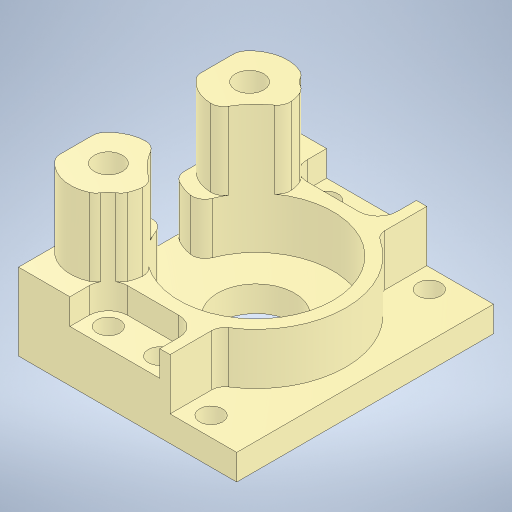
# Autodesk Inventor part: Spring Mount
Saved by Autodesk Inventor 2023.2 (Build 272271000, 271)
## iProperties
Created: 2024-03-24
Part Number: Spring Mount
Material: Nylon 6/6
Document SubType Name: Modeling
Designer: Nathan Cai
Density: 1.13 g/cm^3
Appearance: Nylon 6
Author: Nathan Cai
Autodesk Inventor part; units mm, degrees
ref_plane "YZ Plane" through (0, 0, 0) normal (1, 0, 0) x (0, 1, 0)
ref_plane "XZ Plane" through (0, 0, 0) normal (0, 1, 0) x (-1, 0, 0)
ref_plane "XY Plane" through (0, 0, 0) normal (0, 0, 1) x (1, 0, 0)
sketch "Sketch1" plane through (0, 0, 0) normal (0, 1, 0) x (-1, 0, 0)
  line L0 (-13.4938, 15.875) -> (13.4937, 15.875)
  line L1 (13.4937, 15.875) -> (13.4937, -15.875)
  line L2 (13.4937, -15.875) -> (-13.4938, -15.875)
  line L3 (-13.4938, -15.875) -> (-13.4938, 15.875)
  line L4 (-13.4938, 15.875) -> (13.4937, -15.875) construction
  line L5 (13.4937, 15.875) -> (-13.4938, -15.875) construction
  circle A0 centre (0, 0) radius 4.7625
  circle A1 centre (9.525, 8.7313) radius 6.35 construction
  line L6 (13.4937, 0) -> (-13.4938, 0) construction
  circle A2 centre (9.525, 8.7313) radius 1.7526
  circle A3 centre (9.525, -8.7312) radius 6.35 construction
  circle A4 centre (9.525, -8.7312) radius 1.7526
  dimension "d0" = 26.9875
  dimension "d1" = 31.75
  dimension "d2" = 9.525
  dimension "d3" = 12.7
  dimension "d4" = 3.5052
  dimension "d7" = 8.7312
  dimension "d8" = 3.9688
  constraints: 14 end point, 5 centre point, 4 midpoint, 2 coincident, 2 parallel, 2 symmetric about line, 1 horizontal, 1 perpendicular, 2 other
  measures "d0" distance of L1.end L2.end
  measures "d1" distance of L0.end L1.end
  measures "d2" diameter of A0
  measures "d3" diameter of A1
  measures "d4" diameter of A2
  measures "d7" distance from line of L6 A2.centre
  measures "d8" distance from line of L1 A2.centre
extrude "Extrusion1" add sketch "Sketch1" along normal blind 3.175
sketch "Sketch2" plane through (0, 3.175, 0) normal (0, 1, 0) x (1, 0, 0)
  circle A0 centre (0, 0) radius 9.525
  circle A1 centre (-9.525, 8.7312) radius 1.7526 projected
  circle A2 centre (-9.525, 8.7312) radius 6.35
  line L0 (13.4938, 15.875) -> (-13.4937, 15.875) projected
  line L1 (-13.4937, 15.875) -> (-13.4937, -15.875) projected
  line L2 (-13.4937, -15.875) -> (13.4938, -15.875) projected
  line L3 (13.4938, -15.875) -> (13.4938, 15.875) projected
  circle A3 centre (-9.525, 8.7312) radius 1.7526 projected
  circle A4 centre (-9.525, -8.7313) radius 1.7526 projected
  circle A5 centre (0, 0) radius 4.7625 projected
  circle A6 centre (-9.525, -8.7313) radius 6.35
  point P0 (-13.4937, 13.6882)
  point P1 (-13.4937, 3.7743)
  point P2 (-9.2207, 2.3885)
  point P3 (-3.1798, 8.9786)
  point P4 (-9.2207, -2.3885)
  point P5 (-13.4937, -3.7743)
  point P6 (-13.4937, -13.6882)
  point P7 (-3.1798, -8.9786)
  dimension "d9" = 19.05
  dimension "d10" = 12.7
  dimension "d11" = 12.7
  constraints: 3 centre point, 3 coincident
  measures "d9" diameter of A0
  measures "d10" diameter of A2
  measures "d11" diameter of A6
extrude "Extrusion2" add sketch "Sketch2" along normal blind 6.35 contours A0 A2 L1 L0 L3 L2 A6 | A0 A2 L1 | A6 L1 A0
sketch "Sketch3" plane through (0, 9.525, 0) normal (0, 1, 0) x (1, 0, 0)
  circle A0 centre (-9.525, -8.7313) radius 1.7526 projected
  circle A1 centre (-9.525, -8.7313) radius 4.699
  circle A2 centre (-9.525, 8.7312) radius 1.7526 projected
  circle A3 centre (-9.525, 8.7312) radius 4.699
  arc A4 (-13.4937, 3.7743) -> (-9.2207, 2.3885) centre (-9.525, 8.7312) ccw projected
  arc A5 (-9.2207, -2.3885) -> (-9.2207, 2.3885) centre (0, 0) ccw projected
  line L0 (-13.4937, 15.875) -> (-13.4937, 3.7743) projected
  circle A6 centre (-9.525, 8.7312) radius 1.7526 projected
  line L1 (-13.4937, -3.7743) -> (-13.4937, -15.875) projected
  arc A7 (-9.2207, -2.3885) -> (-13.4937, -3.7743) centre (-9.525, -8.7313) ccw projected
  arc A8 (-9.2207, -2.3885) -> (-9.2207, 2.3885) centre (0, 0) ccw projected
  circle A9 centre (-9.525, -8.7313) radius 1.7526 projected
  arc A10 (-13.4937, 3.7743) -> (-9.2207, 2.3885) centre (-9.525, 8.7312) ccw projected
  line L2 (-13.4937, -15.875) -> (13.4938, -15.875) projected
  line L3 (13.4938, -15.875) -> (13.4938, 15.875) projected
  line L4 (13.4938, 15.875) -> (-13.4937, 15.875) projected
  line L5 (-13.4937, 15.875) -> (-13.4937, 3.7743) projected
  arc A11 (-9.2207, -2.3885) -> (-13.4937, -3.7743) centre (-9.525, -8.7313) ccw projected
  line L6 (-13.4937, -3.7743) -> (-13.4937, -15.875) projected
  line L7 (-13.4937, -15.875) -> (13.4938, -15.875) projected
  line L8 (13.4938, -15.875) -> (13.4938, 15.875) projected
  line L9 (13.4938, 15.875) -> (-13.4937, 15.875) projected
  point P0 (-4.8568, -8.1937)
  point P1 (-8.5843, -4.1274)
  point P2 (-13.4937, -6.2154)
  point P3 (-13.4937, -11.2471)
  point P4 (-13.4937, 11.2471)
  point P5 (-13.4937, 6.2154)
  point P6 (-8.5843, 4.1274)
  point P7 (-4.8568, 8.1937)
  dimension "d14" = 9.398
  dimension "d15" = 9.398
  constraints: 2 centre point, 2 coincident
  measures "d14" diameter of A1
  measures "d15" diameter of A3
extrude "Extrusion3" add sketch "Sketch3" along normal blind 9.525 contours A1 L1 A5 | A5 A3 L0
sketch "Sketch4" plane through (0, 0, 0) normal (0, -1, 0) x (1, 0, 0)
  line L0 (-13.4937, -3.7743) -> (-13.4937, 3.7743) projected
  line L1 (-13.4937, 13.4938) -> (13.4938, 13.4937) construction
  line L2 (13.4938, 15.875) -> (13.4938, -15.875) projected
  line L3 (-13.4937, 15.875) -> (13.4938, 15.875) projected
  circle A0 centre (-11.1125, 13.4938) radius 1.4224
  circle A1 centre (-4.7625, 13.4937) radius 1.4224
  circle A2 centre (1.5875, 13.4937) radius 1.4224
  circle A3 centre (7.9375, 13.4937) radius 1.4224
  line L4 (-13.4937, -3.7743) -> (-13.4937, 3.7743) projected
  line L5 (-13.4937, 0) -> (13.4938, 0) construction
  line L6 (-13.4938, -13.4937) -> (13.4938, -13.4937) construction
  circle A4 centre (-11.1125, -13.4937) radius 1.4224
  circle A5 centre (-4.7625, -13.4937) radius 1.4224
  circle A6 centre (1.5875, -13.4937) radius 1.4224
  circle A7 centre (7.9375, -13.4937) radius 1.4224
  point P0 (0, 0)
  point P1 (-13.4937, 12.8557)
  point P2 (-13.4937, -4.6068)
  point P3 (-13.4937, 4.6068)
  dimension "d19" = 2.3813
  dimension "d20" = 2.8448
  dimension "d21" = 2.3813
  dimension "d24" = 6.35
  constraints: 8 centre point, 6 end point, 6 symmetric about line, 4 point on line, 2 midpoint, 1 horizontal, 1 parallel, 10 other
  measures "d19" distance between parallel lines of L3 L1
  measures "d20" diameter of A0
  measures "d21" distance from line of L0 A0.centre
  measures "d24" distance of A0.centre A1.centre
extrude "Extrusion4" cut sketch "Sketch4" against normal blind 6.35
sketch "Sketch5" plane through (0, 9.525, 0) normal (0, 1, 0) x (1, 0, 0)
  circle A0 centre (7.9375, -13.4937) radius 1.4224 projected
  line L0 (13.4938, -15.875) -> (13.4938, 15.875) projected
  line L1 (13.4938, 0) -> (-13.4937, 0) construction
  line L2 (-13.4937, 15.875) -> (-13.4937, -15.875) projected
  circle A1 centre (1.5875, -13.4937) radius 1.4224 projected
  circle A2 centre (-4.7625, -13.4937) radius 1.4224 projected
  line L3 (1.5875, -13.4937) -> (-4.7625, -13.4937) construction
  line L4 (1.5875, -11.1125) -> (-4.7625, -11.1125)
  line L5 (-4.7625, -15.875) -> (1.5875, -15.875)
  arc A3 (1.5875, -15.875) -> (1.5875, -11.1125) centre (1.5875, -13.4937) ccw
  arc A4 (-4.7625, -11.1125) -> (-4.7625, -15.875) centre (-4.7625, -13.4937) ccw
  line L6 (-13.4937, -15.875) -> (13.4938, -15.875) projected
  line L7 (3.9688, -13.4937) -> (-7.1437, -13.4937) construction
  line L8 (-7.1437, -13.4937) -> (-7.1437, -15.875)
  line L9 (-7.1437, -15.875) -> (3.9688, -15.875)
  line L10 (3.9688, -15.875) -> (3.9688, -13.4937)
  circle A5 centre (1.5875, 13.4937) radius 1.4224
  circle A6 centre (-4.7625, 13.4937) radius 1.4224
  line L11 (1.5875, 13.4937) -> (-4.7625, 13.4937) construction
  line L12 (1.5875, 11.1125) -> (-4.7625, 11.1125)
  line L13 (-4.7625, 15.875) -> (1.5875, 15.875)
  arc A7 (1.5875, 11.1125) -> (1.5875, 15.875) centre (1.5875, 13.4937) ccw
  arc A8 (-4.7625, 15.875) -> (-4.7625, 11.1125) centre (-4.7625, 13.4937) ccw
  line L14 (3.9688, 13.4937) -> (-7.1437, 13.4937) construction
  line L15 (-7.1437, 13.4937) -> (-7.1437, 15.875)
  line L16 (-7.1437, 15.875) -> (3.9688, 15.875)
  line L17 (3.9688, 15.875) -> (3.9688, 13.4937)
  point P0 (0, 0)
  point P1 (-1.5875, -13.4937)
  point P2 (-1.5875, 13.4937)
  constraints: 34 end point, 11 symmetric about line, 9 point on circle, 6 centre point, 5 tangent, 3 midpoint, 3 parallel, 2 horizontal, 2 point on line, 1 perpendicular, 4 other
extrude "Extrusion5" cut sketch "Sketch5" along normal blind 25.4 and the other way blind 3.175 contours A1 | A2 | A3 L5 A4 L4 | L10 L6 A3 | A4 L6 L8 | A5 | A6 | L12 A8 L13 A7 | A7 L16 L17 | L15 L16 A8
fillet "Fillet3" radius 1.5875 16 edges at (-4.8568, 14.2875, 8.1937) (-8.5843, 14.2875, 4.1274) (-7.0071, 14.2875, -12.6987) (-5.5575, 14.2875, -11.2491) (-13.4937, 14.2875, -11.2471) (-4.8568, 14.2875, -8.1937) (-8.5843, 14.2875, -4.1274) (-7.0071, 14.2875, 12.6987) (-5.5575, 14.2875, 11.2491) (-13.4937, 14.2875, 11.2471) (-13.4937, 14.2875, 6.2154) (-13.4937, 14.2875, -6.2154) (-9.2207, 6.35, 2.3885) (-9.2207, 6.35, -2.3885) (-13.4937, 6.35, -3.7743) (-13.4937, 6.35, 3.7743)
sketch "Sketch6" plane through (0, 9.525, 0) normal (0, 1, 0) x (1, 0, 0)
  line L0 (13.4938, -15.875) -> (13.4938, 15.875) projected
  circle A0 centre (0, 0) radius 11.1125
  line L1 (3.9688, -15.875) -> (13.4938, -15.875) projected
  line L2 (5.247, -15.875) -> (5.247, -9.7958)
  line L3 (0, 0) -> (11.1125, 0) construction
  line L4 (3.9688, -13.4937) -> (3.9688, -15.875) projected
  line L5 (5.247, 15.875) -> (5.247, 9.7958)
  line L6 (3.9688, 15.875) -> (3.9688, 13.4937) projected
  arc A1 (1.5875, 11.1125) -> (3.9688, 13.4937) centre (1.5875, 13.4937) ccw projected
  line L7 (1.5875, 11.1125) -> (-4.7625, 11.1125) projected
  arc A2 (-5.923, 11.4144) -> (-4.7625, 11.1125) centre (-4.7625, 13.4937) ccw projected
  arc A3 (-5.2537, 10.69) -> (-5.923, 11.4144) centre (-6.6967, 10.0282) ccw projected
  arc A4 (-4.8527, 9.2314) -> (-5.2537, 10.69) centre (-9.525, 8.7312) ccw projected
  arc A5 (-5.5124, 7.7678) -> (-4.8527, 9.2314) centre (-6.4312, 9.0624) ccw projected
  arc A6 (-5.5124, -7.7678) -> (-5.5124, 7.7678) centre (0, 0) ccw projected
  arc A7 (-4.8527, -9.2314) -> (-5.5124, -7.7678) centre (-6.4312, -9.0624) ccw projected
  arc A8 (-5.2537, -10.69) -> (-4.8527, -9.2314) centre (-9.525, -8.7313) ccw projected
  arc A9 (-5.923, -11.4144) -> (-5.2537, -10.69) centre (-6.6967, -10.0282) ccw projected
  arc A10 (-4.7625, -11.1125) -> (-5.923, -11.4144) centre (-4.7625, -13.4937) ccw projected
  line L8 (-4.7625, -11.1125) -> (1.5875, -11.1125) projected
  arc A11 (3.9688, -13.4937) -> (1.5875, -11.1125) centre (1.5875, -13.4937) ccw projected
  line L9 (3.9688, -13.4937) -> (3.9688, -15.875) projected
  line L10 (3.9688, -15.875) -> (13.4938, -15.875) projected
  line L11 (13.4938, -15.875) -> (13.4938, 15.875) projected
  line L12 (13.4938, 15.875) -> (3.9688, 15.875) projected
  dimension "d42" = 22.225
  dimension "d43" = 1.2782
  constraints: 6 end point, 2 perpendicular, 2 point on circle, 2 symmetric about line, 1 centre point, 1 coincident, 1 point on line
  measures "d42" diameter of A0
  measures "d43" distance between parallel lines of L4 L2
extrude "Extrusion6" cut sketch "Sketch6" against normal blind 6.35 contours L1 L2 A0 L5 L12 L0
fillet "Fillet4" radius 1.5875 2 edges at (5.247, 6.35, -9.7958) (5.247, 6.35, 9.7958)
equation "\"d11\" = d10"
body "Solid1"
